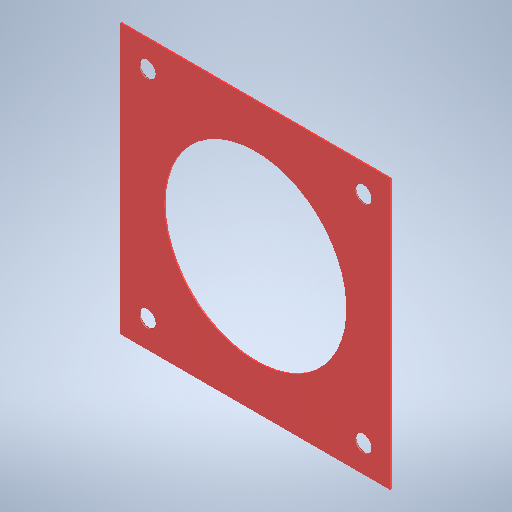
# Autodesk Inventor part: zylinderfussdichtung
Saved by Autodesk Inventor 2025 (Build 290162010, 162A)
## iProperties
Created: 2024-04-30
Part Number: zylinderfussdichtung
Material: Generisch
Document SubType Name: Modeling
Designer: ffogue
Density: 1 g/cm^3
Appearance: Light Red
Author: ffogue
Autodesk Inventor part; units mm, degrees
ref_plane "YZ Plane" through (0, 0, 0) normal (1, 0, 0) x (0, 1, 0)
ref_plane "XZ Plane" through (0, 0, 0) normal (0, 1, 0) x (-1, 0, 0)
ref_plane "XY Plane" through (0, 0, 0) normal (0, 0, 1) x (1, 0, 0)
sketch "Skizze1" plane through (0, 0, 0) normal (0, 1, 0) x (-1, 0, 0)
  line L0 (-20, 20) -> (20, 20)
  line L1 (20, 20) -> (20, -20)
  line L2 (20, -20) -> (-20, -20)
  line L3 (-20, -20) -> (-20, 20)
  circle A0 centre (0, 0) radius 13.5
  dimension "d0" = 40
  dimension "d1" = 40
  dimension "d2" = 27
  dimension "d16" = 20
  constraints: 8 end point, 2 parallel, 1 centre point, 1 coincident, 1 horizontal, 1 perpendicular
  measures "d0" distance of L1.end L2.end
  measures "d1" distance of L0.end L1.end
  measures "d2" diameter of A0
  measures "d16" distance from line of L2 point (0, 0)
extrude "Extrusion1" add sketch "Skizze1" against normal blind 0.2
sketch "Skizze2" plane through (0, -0.2, 0) normal (0, -1, 0) x (1, 0, 0)
  point P0 (0, 0)
  point P1 (-16, -16)
  point P2 (-16, 16)
  point P3 (16, -16)
  point P4 (16, 16)
  dimension "d12" = 32
  dimension "d13" = 16
  dimension "d14" = 32
  dimension "d15" = 16
  constraints: 2 horizontal alignment, 2 vertical alignment
  measures "d12" distance of point (16, 16) point (16, -16)
  measures "d13" horizontal distance of point (16, -16) point (0, 0)
  measures "d14" distance of point (-16, 16) point (16, 16)
  measures "d15" horizontal distance of point (0, 0) point (-16, 16)
hole "Bohrung1" at (-16, -0.2, -16) at (-16, -0.2, 16) at (16, -0.2, -16) at (16, -0.2, 16) direction (0, 1, 0) diameter 2.459 depth 0.2 thread size "M3x0.5" class "6H" standard "ISO Metric profile"
